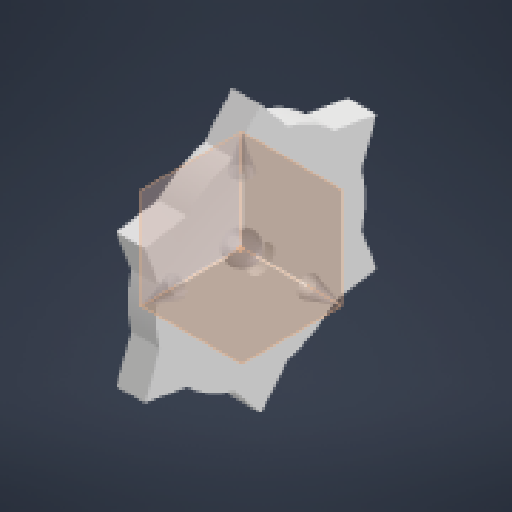
# Autodesk Inventor part: Vertical Spinner Weapon V3
Saved by Autodesk Inventor 2026.2 (Build 302298000, 298)
## iProperties
Created: 2023-08-18
Part Number: Vertical Spinner Weapon V3
Material: Generic
Document SubType Name: Modeling
Designer: vandj
Density: 1 g/cm^3
Appearance: Default
Mass: 70.3924 g
Surface Area: 175.698 cm^2
Volume: 70.3924 cm^3
Author: vandj
Autodesk Inventor part; units mm, degrees
ref_plane "YZ Plane" through (0, 0, 0) normal (1, 0, 0) x (0, 1, 0)
ref_plane "XZ Plane" through (0, 0, 0) normal (0, 1, 0) x (-1, 0, 0)
ref_plane "XY Plane" through (0, 0, 0) normal (0, 0, 1) x (1, 0, 0)
sketch "Sketch 1" plane through (0, 0, 0) normal (1, 0, 0) x (0, 1, 0)
  circle A0 centre (0, 0) radius 2.5
  circle A1 centre (0, 0) radius 25
  point P0 (1.2916, -31.2195)
  point P1 (0, 30.3272)
  point P2 (-0.1255, 30.3272)
  point P3 (0, -30.3272)
  point P4 (0.1231, -30.3272)
  point P5 (-1.2948, 31.2193)
  point P6 (0.0032, -40.9065)
  point P7 (0, -40.9065)
  point P8 (-1.4137, 30.3272)
  dimension "d22" = 5
  dimension "d51" = 50
  constraints: 2 centre point, 2 coincident
  measures "d22" diameter of A0
  measures "d51" diameter of A1
extrude "Interface" add sketch "Sketch 1" along normal blind 15
sketch "Sketch9" plane through (0, 0, 0) normal (-1, 0, 0) x (0, 0, 1)
  circle A0 centre (0, 0) radius 2.5 projected
  circle A1 centre (0, 0) radius 3.75
  dimension "d32" = 7.5
  constraints: 1 centre point, 1 coincident
  measures "d32" diameter of A1
extrude "Shaft Hole" cut sketch "Sketch9" against normal blind 28.1375
sketch "Sketch10" plane through (15, 0, 0) normal (1, 0, 0) x (0, 0, -1)
  circle A0 centre (0, 0) radius 3.75 projected
  circle A1 centre (0, 0) radius 7
  dimension "d35" = 14
  constraints: 1 centre point, 1 coincident
  measures "d35" diameter of A1
extrude "Bearing Hole" cut sketch "Sketch10" against normal blind 5
sketch "EDIT WEAPON SKETCH" plane through (0, 0, 0) normal (1, 0, 0) x (0, 1, 0)
  circle A0 centre (0, 0) radius 25 projected
  circle A1 centre (0, 0) radius 25 projected
  circle A2 centre (0, 0) radius 70
  line L0 (80.6762, 135.1886) -> (80.6762, 42.6083) construction
  line L1 (80.6762, 42.6083) -> (64.461, 42.6083) construction
  line L2 (64.461, 42.6083) -> (64.461, 135.1886) construction
  line L3 (64.461, 135.1886) -> (80.6762, 135.1886) construction
  line L4 (-69.9999, -0.1091) -> (-52.7296, -14.3724)
  line L5 (-69.9999, -0.1091) -> (-52.7886, 14.1542)
  line L6 (-34.9055, -60.6762) -> (-13.918, -52.8514)
  line L7 (-34.9055, -60.6762) -> (-38.6522, -38.6392)
  line L8 (35.0944, -60.5672) -> (38.8116, -38.479)
  line L9 (35.0944, -60.5672) -> (14.1364, -52.7934)
  line L10 (69.9999, 0.1091) -> (52.7296, 14.3724)
  line L11 (69.9999, 0.1091) -> (52.7886, -14.1542)
  line L12 (34.9055, 60.6762) -> (13.918, 52.8514)
  line L13 (34.9055, 60.6762) -> (38.6522, 38.6392)
  line L14 (-35.0944, 60.5672) -> (-38.8116, 38.479)
  line L15 (-35.0944, 60.5672) -> (-14.1364, 52.7934)
  circle A3 centre (0, 0) radius 3.75 projected
  arc A4 (-52.7296, -14.3724) -> (-38.6522, -38.6392) centre (0, 0) ccw
  arc A5 (-38.8116, 38.479) -> (-52.7886, 14.1542) centre (0, 0) ccw
  arc A6 (13.918, 52.8514) -> (-14.1364, 52.7934) centre (0, 0) ccw
  arc A7 (52.7296, 14.3724) -> (38.6522, 38.6392) centre (0, 0) ccw
  arc A8 (-13.918, -52.8514) -> (14.1364, -52.7934) centre (0, 0) ccw
  arc A9 (38.8116, -38.479) -> (52.7886, -14.1542) centre (0, 0) ccw
  dimension "d60" = 140
  dimension "d64" = 14.2633
  dimension "d65" = 14.2633
  dimension "d68" = 360
  dimension "d70" = 0
  dimension "d71" = 0
  dimension "d72" = 0
  constraints: 24 end point, 12 point on circle, 6 centre point, 6 point on line, 1 coincident, 36 other
  measures "d64" vertical distance of L4.start L4.end
  measures "d65" vertical distance of L4.start L5.end
  measures "d70" distance of A6.end L15.end
  measures "d71" distance of A7.end L13.end
  measures "d72" distance of L11.end A9.end
extrude "EDIT WEAPON SHAPE" add sketch "EDIT WEAPON SKETCH" along normal up to surface (15 mm away) contours L11 A9 L8 L9 A8 L6 L7 A4 L4 L5 A5 L14 L15 A6 L12 L13 A7 L10
sketch "Sketch12" plane through (0, 0, 0) normal (-1, 0, 0) x (0, 0, 1)
  point P0 (0, 0)
body "Solid1"
